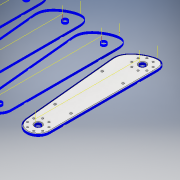
# Autodesk Inventor part: Sigma106_tibiaplate_design
Saved by Autodesk Inventor 2018 (Build 220112000, 112)
## iProperties
Created: 2016-05-06
Part Number: Sigma106_tibiaplate_design
Material: Aluminum 2014-T4
Document SubType Name: Modeling
Designer: steve
Density: 2.8 g/cm^3
Appearance: Satin
Mass: 44.479 g
Surface Area: 124.066 cm^2
Volume: 15.8853 cm^3
Vendor: Rhoban
Sheet Metal Rule: Default_mm
Author: steve
Autodesk Inventor part; units mm, degrees
ref_plane "YZ Plane" through (0, 0, 0) normal (1, 0, 0) x (0, 1, 0)
ref_plane "XZ Plane" through (0, 0, 0) normal (0, 1, 0) x (-1, 0, 0)
ref_plane "XY Plane" through (0, 0, 0) normal (0, 0, 1) x (1, 0, 0)
sketch "Sketch2" plane through (0, 0, 0) normal (0, 0, 1) x (1, 0, 0)
  circle A0 centre (0, 0) radius 14 construction
  line L0 (0, -78.1672) -> (0, 269.7416) construction
  line L1 (0, -28.466) -> (0, 220.0403) construction
  circle A1 centre (0, 140) radius 14 construction
  line L2 (-14, 0) -> (-14, 140)
  line L3 (14, 140) -> (14, 0)
  arc A2 (14, 140) -> (-14, 140) centre (0, 140) ccw
  arc A3 (-14, 0) -> (14, 0) centre (0, 0) ccw
  circle A4 centre (0, 140) radius 5.05
  circle A5 centre (0, 0) radius 5.05
  dimension "d0" = 28
  dimension "d1" = 28
  dimension "d2" = 140
  dimension "d3" = 10.1
  dimension "d4" = 10.1
  measures "d0" diameter of A0
  measures "d1" diameter of A1
  measures "d2" distance of point (0, 0) A1.centre
  measures "d3" diameter of A4
  measures "d4" diameter of A5
extrude "Plate1" add sketch "Sketch2" along normal blind 3
sketch "Sketch3" plane through (0, 0, 3) normal (0, 0, 1) x (1, 0, 0)
  circle A0 centre (0, 0) radius 11 construction
  circle A1 centre (0, 140) radius 11 construction
  circle A2 centre (0, 140) radius 8.5 construction
  circle A3 centre (0, 140) radius 5.05 construction
  line L0 (0, 0) -> (12.8086, 5.3055) construction
  line L1 (0, 0) -> (13.8639, 0) construction
  line L2 (12.8086, 5.3055) -> (12.5617, 5.9016) construction
  line L3 (0, 140) -> (16.0819, 146.6613) construction
  line L4 (0, 140) -> (17.4069, 140) construction
  line L5 (-9, 137.5621) -> (-9, -33.762) construction
  line L6 (9, -33.762) -> (9, 143.7894) construction
  line L7 (-14, 0) -> (-14, 140) construction
  line L8 (14, 140) -> (14, 0) construction
  line L9 (-30.9821, 105) -> (51.5896, 105) construction
  line L10 (-30.9821, 35) -> (48.2288, 35) construction
  point P0 (10.1627, 4.2095)
  point P1 (4.2095, 10.1627)
  point P2 (-4.2095, 10.1627)
  point P3 (-10.1627, 4.2095)
  point P4 (10.1627, 144.2095)
  point P5 (4.2095, 150.1627)
  point P6 (-4.2095, 150.1627)
  point P7 (-10.1627, 144.2095)
  point P8 (-10.1627, 135.7905)
  point P9 (-4.2095, 129.8373)
  point P10 (4.2095, 129.8373)
  point P11 (10.1627, 135.7905)
  point P12 (-10.1627, -4.2095)
  point P13 (-4.2095, -10.1627)
  point P14 (4.2095, -10.1627)
  point P15 (10.1627, -4.2095)
  dimension "d6" = 22
  dimension "d8" = 22
  dimension "d14" = 22.5
  dimension "d17" = 360
  dimension "d23" = 22.5
  dimension "d26" = 360
  dimension "d29" = 5
  dimension "d30" = 5
  dimension "d31" = 35
  dimension "d32" = 35
  constraints: 18 end point, 4 horizontal, 2 coincident, 2 equal length, 2 point on line, 1 centre point, 1 concentric, 1 perpendicular, 1 vertical, 25 other
  measures "d14" angle of L1 L0
  measures "d23" angle of L4 L3
  measures "d29" distance between parallel lines of L7 L5
  measures "d30" distance between parallel lines of L8 L6
  measures "d31" distance from line of L9 point (0, 140)
  measures "d32" distance from line of L10 point (0, 0)
hole "Hole1" at (10.1627, 4.2095, 3) at (4.2095, 10.1627, 3) at (-4.2095, 10.1627, 3) at (-10.1627, 4.2095, 3) at (10.1627, 144.2095, 3) at (4.2095, 150.1627, 3) at (-4.2095, 150.1627, 3) at (-10.1627, 144.2095, 3) at (10.1627, 135.7905, 3) at (4.2095, 129.8373, 3) at (-4.2095, 129.8373, 3) at (-10.1627, 135.7905, 3) at (10.1627, -4.2095, 3) at (4.2095, -10.1627, 3) at (-4.2095, -10.1627, 3) at (-10.1627, -4.2095, 3) direction (0, 0, -1) diameter 2.5 end through all
sketch "Sketch4" plane through (0, 0, 3) normal (0, 0, 1) x (1, 0, 0)
  line L0 (-9, 137.5621) -> (-9, -33.762) construction
  line L1 (-30.9821, 105) -> (51.5896, 105) construction
  line L2 (-30.9821, 35) -> (48.2288, 35) construction
  line L3 (9, -33.762) -> (9, 143.7894) construction
  point P0 (0, 0)
  point P1 (-9, 105)
  point P2 (9, 105)
  point P3 (-9, 35)
  point P4 (9, 35)
  constraints: 8 point on line
hole "Hole2" at (-9, 105, 3) at (9, 105, 3) at (-9, 35, 3) at (9, 35, 3) direction (0, 0, -1) diameter 3 end through all
sketch "Sketch5" plane through (0, 0, 0) normal (0, 0, -1) x (-1, 0, 0)
  line L0 (13.9366, -1.3313) -> (25.9336, 124.254)
  circle A0 centre (9, 35) radius 1.5 projected
  circle A1 centre (9, 105) radius 1.5 projected
  circle A2 centre (-9, 105) radius 1.5 projected
  circle A3 centre (-9, 35) radius 1.5 projected
  circle A4 centre (4.2095, -10.1627) radius 1.25 projected
  circle A5 centre (-10.1627, -4.2095) radius 1.25 projected
  circle A6 centre (4.2095, 129.8373) radius 1.25 projected
  circle A7 centre (-10.1627, 135.7905) radius 1.25 projected
  circle A8 centre (4.2095, 150.1627) radius 1.25 projected
  circle A9 centre (-10.1627, 144.2095) radius 1.25 projected
  circle A10 centre (4.2095, 10.1627) radius 1.25 projected
  circle A11 centre (-10.1627, 4.2095) radius 1.25 projected
  circle A12 centre (-4.2095, 10.1627) radius 1.25 projected
  circle A13 centre (10.1627, 4.2095) radius 1.25 projected
  circle A14 centre (-4.2095, 150.1627) radius 1.25 projected
  circle A15 centre (10.1627, 144.2095) radius 1.25 projected
  circle A16 centre (-4.2095, 129.8373) radius 1.25 projected
  circle A17 centre (10.1627, 135.7905) radius 1.25 projected
  circle A18 centre (-4.2095, -10.1627) radius 1.25 projected
  circle A19 centre (10.1627, -4.2095) radius 1.25 projected
  circle A20 centre (0, 0) radius 5.05 projected
  circle A21 centre (0, 140) radius 5.05 projected
  line L1 (14, 0) -> (14, 140) projected
  arc A22 (14, 140) -> (-14, 140) centre (0, 140) ccw projected
  line L2 (-14, 140) -> (-14, 0) projected
  arc A23 (-14, 0) -> (14, 0) centre (0, 0) ccw projected
  spline S0 degree 4 poles (25.9336, 124.254) (26.6284, 131.5272) (28.018, 146.0735) (-14, 167.0982) (-14, 149.0327) (-14, 140) knots 0 0 0 0 0 0.5 1 1 1 1 1
  constraints: 2 end point, 1 point on circle, 1 tangent, 1 vertical, 3 other
extrude "Extrusion1" add sketch "Sketch5" against normal blind 3
sketch "Sketch6" plane through (0, 0, 3) normal (0, 0, 1) x (1, 0, 0)
  circle A0 centre (-9, 35) radius 1.5 construction
  circle A1 centre (-9, 105) radius 1.5 construction
  circle A2 centre (9, 105) radius 1.5 construction
  circle A3 centre (9, 35) radius 1.5 construction
  circle A4 centre (-4.2095, -10.1627) radius 1.25 construction
  circle A5 centre (10.1627, -4.2095) radius 1.25 construction
  circle A6 centre (-4.2095, 129.8373) radius 1.25 construction
  circle A7 centre (10.1627, 135.7905) radius 1.25 construction
  circle A8 centre (-4.2095, 150.1627) radius 1.25 construction
  circle A9 centre (10.1627, 144.2095) radius 1.25 construction
  circle A10 centre (-4.2095, 10.1627) radius 1.25 construction
  circle A11 centre (10.1627, 4.2095) radius 1.25 construction
  circle A12 centre (4.2095, 10.1627) radius 1.25 construction
  circle A13 centre (-10.1627, 4.2095) radius 1.25 construction
  circle A14 centre (4.2095, 150.1627) radius 1.25 construction
  circle A15 centre (-10.1627, 144.2095) radius 1.25 construction
  circle A16 centre (4.2095, 129.8373) radius 1.25 construction
  circle A17 centre (-10.1627, 135.7905) radius 1.25 construction
  circle A18 centre (4.2095, -10.1627) radius 1.25 construction
  circle A19 centre (-10.1627, -4.2095) radius 1.25 construction
  circle A20 centre (0, 0) radius 5.05 construction
  circle A21 centre (0, 140) radius 5.05 construction
  line L0 (-25.9336, 124.254) -> (-13.9366, -1.3313) construction
  arc A22 (-13.9366, -1.3313) -> (14, 0) centre (0, 0) ccw construction
  line L1 (14, 140) -> (14, 0) construction
  circle A23 centre (9, 105) radius 1.5 construction
  line L2 (9, 105) -> (-38.107, 105) construction
  circle A24 centre (9, 35) radius 1.5 construction
  line L3 (9, 35) -> (-44.0187, 35) construction
  line L4 (-24.3019, 159.7512) -> (-5.7807, -34.1287) construction
  line L5 (-25.9336, 124.254) -> (-13.9366, -1.3313) construction
  point P0 (-19.0715, 105)
  point P1 (-12.3845, 35)
  dimension "d49" = 5
  constraints: 6 end point, 4 point on line, 2 horizontal, 1 parallel, 1 other
  measures "d49" distance between parallel lines of L0 L4
hole "Hole3" at (-19.0715, 105, 3) at (-12.3845, 35, 3) direction (0, 0, -1) diameter 3 end through all
sketch "Sketch7" plane through (0, 0, 3) normal (0, 0, 1) x (1, 0, 0)
  circle A0 centre (-9, 105) radius 1.5 projected
  circle A1 centre (-9, 35) radius 1.5 projected
  point P0 (0, 0)
extrude "Extrusion2" add sketch "Sketch7" against normal blind 3
equation "\"d2\" = Sigma_plate_axis_to_axis"
equation "\"d3\" = Sigma_plate_axis_hole"
equation "\"d4\" = Sigma_plate_axis_hole"
equation "\"d6\" = Sigma_horn_holes1"
equation "\"d8\" = Sigma_horn_holes1"
equation "\"d38\" = Thickness"
equation "\"d45\" = Thickness"
equation "\"d55\" = Thickness"
equation "\"d59\" = Thickness"
equation "\"BendRadius\" = Thickness"
equation "\"BendReliefWidth\" = Thickness"
equation "\"BendReliefDepth\" = 0.5 * Thickness"
equation "\"CornerReliefSize\" = 4 * Thickness"
equation "\"MinimumRemnant\" = 2 * Thickness"
equation "\"TransitionRadius\" = BendRadius"
equation "\"JacobiRadiusSize\" = BendRadius"
equation "\"GapSize\" = Thickness"
equation "\"Sigma_plate_axis_to_axis\" = 140"
equation "\"tolerance\" = 0.1"
equation "\"d5\" = BendRadius"
equation "\"Sigma_horn_holes1\" = 22"
equation "\"Sigma_horn_holes2\" = 17"
equation "\"Sigma_plate_axis_hole\" = 10.1"
equation "\"Thickness\" = 3"
body "Solid1"
